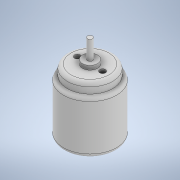
# Autodesk Inventor part: MOTOR
Saved by Autodesk Inventor 2022 (Build 260153070, 153G)
## iProperties
Created: 2021-10-27
Part Number: MOTOR
Material: Generic
Document SubType Name: Modeling
Designer: a laptop
Density: 1 g/cm^3
Appearance: Default
Mass: 8.41914 g
Surface Area: 23.8486 cm^2
Volume: 8.41914 cm^3
Author: a laptop
Autodesk Inventor part; units mm, degrees
ref_plane "YZ Plane" through (0, 0, 0) normal (1, 0, 0) x (0, 1, 0)
ref_plane "XZ Plane" through (0, 0, 0) normal (0, 1, 0) x (-1, 0, 0)
ref_plane "XY Plane" through (0, 0, 0) normal (0, 0, 1) x (1, 0, 0)
sketch "Sketch3" plane through (0, 0, 0) normal (0, 0, 1) x (1, 0, 0)
  line L0 (0, 0) -> (6.25, 0)
  line L1 (6.25, 0) -> (6.25, -2)
  line L2 (1.5, 25) -> (7.5, 25)
  line L3 (7.5, 25) -> (7.5, 26.6)
  line L4 (10.5, 21) -> (10.5, -2)
  line L5 (6.25, -2) -> (10.5, -2)
  line L6 (7.5, 26.6) -> (9.5, 26.6)
  line L7 (9.5, 26.6) -> (9.5, 34.6)
  line L8 (9.5, 34.6) -> (10.5, 34.6)
  line L9 (10.5, 34.6) -> (10.5, 21)
  line L10 (1.5, 25) -> (1.5, 21)
  line L11 (1.5, 21) -> (0, 21)
  line L12 (0, 21) -> (0, 0)
  dimension "d5" = 4.25
  dimension "d7" = 1.6
  dimension "d10" = 1
  dimension "d13" = 2
  dimension "d16" = 3
  dimension "d17" = 8
  dimension "d18" = 25
  dimension "d19" = 1.5
  dimension "d20" = 4
  dimension "d21" = 10.5
  dimension "d23" = 6.25
  constraints: 26 end point, 6 perpendicular, 3 horizontal, 1 collinear, 1 vertical
  measures "d5" distance of L1.end L4.end
  measures "d7" distance of L2.end L3.end
  measures "d10" distance of L7.end L8.end
  measures "d13" distance of L0.end L1.end
  measures "d16" distance from line of L3.end L9
  measures "d17" distance between parallel lines of L8 L6
  measures "d18" vertical distance of L0.start L2.start
  measures "d19" distance of L10.end L11.end
  measures "d20" distance of L2.start L10.end
  measures "d21" distance between parallel lines of L4 L12
  measures "d23" distance of L0.start L0.end
revolve "Revolution1" add sketch "Sketch3" angle 360 about axis through (10.5, 21, 0) along (0, -1, 0)
fillet "Fillet1" radius 1.5 3 edges at (19.5, 25, 0) (21, 0, 0) (21, 21, 0)
sketch "Sketch4" plane through (10.5, 25, 0) normal (0, 1, 0) x (1, 0, 0)
  circle A0 centre (0, 0) radius 1 projected
  circle A1 centre (0, 0) radius 5 construction
  circle A2 centre (-5, 0) radius 1.15
  line L0 (-14.7, 0) -> (14.7, 0) projected
  circle A3 centre (5, 0) radius 1.15
  point P0 (-10.5, 0)
  dimension "d24" = 10
  dimension "d25" = 2.3
  dimension "d28" = 360
  constraints: 2 centre point, 1 coincident, 1 horizontal alignment, 1 point on line, 7 other
  measures "d25" diameter of A2
extrude "Extrusion2" cut sketch "Sketch4" against normal blind 2 contours L0 A2 | A2 L0 | A3 L0 | L0 A3
sketch "Sketch5" plane through (10.5, 34.6, 0) normal (0, 1, 0) x (1, 0, 0)
  circle A0 centre (0, 0) radius 1 projected
  point P0 (-10.5, 0)
extrude "Extrusion3" cut sketch "Sketch5" against normal blind 0.5
body "Solid2"
